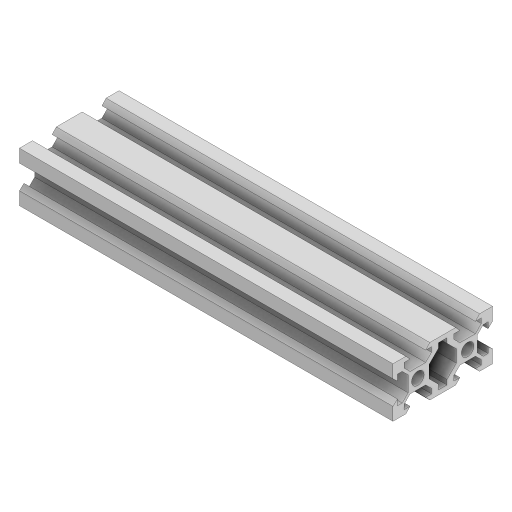
# Autodesk Inventor part: VSLOT
Saved by Autodesk Inventor 2024 (Build 280153000, 153)
## iProperties
Created: 2024-05-16
Part Number: VSLOT
Material: Generic
Document SubType Name: Modeling
Designer: Jhuliams
Density: 1 g/cm^3
Appearance: Default
Author: Jhuliams
Autodesk Inventor part; units mm, degrees
ref_plane "YZ Plane" through (0, 0, 0) normal (1, 0, 0) x (0, 1, 0)
ref_plane "XZ Plane" through (0, 0, 0) normal (0, 1, 0) x (-1, 0, 0)
ref_plane "XY Plane" through (0, 0, 0) normal (0, 0, 1) x (1, 0, 0)
sketch "Sketch1" plane through (0, 0, 0) normal (1, 0, 0) x (0, 1, 0)
  line L0 (10, 20) -> (-10, 20)
  line L1 (-10, 20) -> (-10, -20)
  line L2 (-10, -20) -> (10, -20)
  line L3 (10, -20) -> (10, 20)
  line L4 (10, 20) -> (-10, -20) construction
  line L5 (-10, 20) -> (10, -20) construction
  line L6 (0, -20) -> (0, -10) construction
  circle A0 centre (0, -10) radius 2.5
  line L7 (10, 0) -> (0, 0) construction
  circle A1 centre (0, 10) radius 2.5
  line L8 (0, 20) -> (0, 18.2) construction
  line L9 (0, 18.2) -> (3.125, 18.2)
  line L10 (0, 18.2) -> (0, 13.9)
  line L11 (0, 20) -> (4.8, 20)
  line L12 (4.8, 20) -> (3.125, 18.2)
  line L13 (0, 18.2) -> (5.5, 18.2)
  line L14 (0, 13.9) -> (3.125, 13.9)
  line L15 (5.5, 18.2) -> (5.5, 16.275)
  line L16 (3.125, 13.9) -> (5.5, 16.275)
  line L17 (3.125, 13.9) -> (8.7353, 13.9) construction
  line L18 (0, 18.2) -> (-3.125, 18.2)
  line L19 (0, 20) -> (-4.8, 20)
  line L20 (-4.8, 20) -> (-3.125, 18.2)
  line L21 (0, 18.2) -> (-5.5, 18.2)
  line L22 (0, 13.9) -> (-3.125, 13.9)
  line L23 (-5.5, 18.2) -> (-5.5, 16.275)
  line L24 (-3.125, 13.9) -> (-5.5, 16.275)
  line L25 (10, 10) -> (8.2, 10) construction
  line L26 (8.2, 10) -> (8.2, 6.875)
  line L27 (8.2, 10) -> (3.9, 10)
  line L28 (10, 10) -> (10, 5.2)
  line L29 (10, 5.2) -> (8.2, 6.875)
  line L30 (8.2, 10) -> (8.2, 4.5)
  line L31 (3.9, 10) -> (3.9, 6.875)
  line L32 (8.2, 4.5) -> (6.275, 4.5)
  line L33 (3.9, 6.875) -> (6.275, 4.5)
  line L34 (3.9, 13.125) -> (6.275, 15.5)
  line L35 (8.2, 10) -> (8.2, 15.5)
  line L36 (8.2, 15.5) -> (6.275, 15.5)
  line L37 (8.2, 10) -> (8.2, 13.125)
  line L38 (10, 10) -> (10, 14.8)
  line L39 (10, 14.8) -> (8.2, 13.125)
  line L40 (3.9, 10) -> (3.9, 13.125)
  line L41 (0, 10) -> (10, 10) construction
  line L42 (-3.9, 10) -> (-3.9, 13.125)
  line L43 (-3.9, 13.125) -> (-6.275, 15.5)
  line L44 (-8.2, 10) -> (-8.2, 15.5)
  line L45 (-8.2, 15.5) -> (-6.275, 15.5)
  line L46 (-10, 14.8) -> (-8.2, 13.125)
  line L47 (-3.9, 10) -> (-3.9, 6.875)
  line L48 (-3.9, 6.875) -> (-6.275, 4.5)
  line L49 (-8.2, 4.5) -> (-6.275, 4.5)
  line L50 (-8.2, 10) -> (-8.2, 4.5)
  line L51 (-10, 5.2) -> (-8.2, 6.875)
  line L52 (0, -20) -> (0, -18.2) construction
  line L53 (0, -18.2) -> (3.125, -18.2)
  line L54 (0, -18.2) -> (0, -13.9)
  line L55 (0, -20) -> (4.8, -20)
  line L56 (4.8, -20) -> (3.125, -18.2)
  line L57 (0, -18.2) -> (5.5, -18.2)
  line L58 (0, -13.9) -> (3.125, -13.9)
  line L59 (5.5, -18.2) -> (5.5, -16.275)
  line L60 (3.125, -13.9) -> (5.5, -16.275)
  line L61 (3.125, -13.9) -> (8.7353, -13.9) construction
  line L62 (-3.125, -13.9) -> (-5.5, -16.275)
  line L63 (0, -18.2) -> (-5.5, -18.2)
  line L64 (-5.5, -18.2) -> (-5.5, -16.275)
  line L65 (0, -18.2) -> (-3.125, -18.2)
  line L66 (0, -20) -> (-4.8, -20)
  line L67 (-4.8, -20) -> (-3.125, -18.2)
  line L68 (0, -13.9) -> (-3.125, -13.9)
  line L69 (8.2, -10) -> (8.2, -13.125)
  line L70 (3.9, -10) -> (3.9, -13.125)
  line L71 (3.9, -13.125) -> (6.275, -15.5)
  line L72 (10, -10) -> (10, -14.8)
  line L73 (8.2, -10) -> (8.2, -15.5)
  line L74 (8.2, -15.5) -> (6.275, -15.5)
  line L75 (10, -14.8) -> (8.2, -13.125)
  line L76 (3.9, -10) -> (3.9, -6.875)
  line L77 (3.9, -6.875) -> (6.275, -4.5)
  line L78 (8.2, -4.5) -> (6.275, -4.5)
  line L79 (8.2, -10) -> (3.9, -10)
  line L80 (8.2, -10) -> (8.2, -6.875)
  line L81 (8.2, -10) -> (8.2, -4.5)
  line L82 (10, -5.2) -> (8.2, -6.875)
  line L83 (10, -10) -> (10, -5.2)
  line L84 (10, -10) -> (8.2, -10) construction
  line L85 (-10, -14.8) -> (-8.2, -13.125)
  line L86 (-8.2, -10) -> (-8.2, -15.5)
  line L87 (-8.2, -15.5) -> (-6.275, -15.5)
  line L88 (-3.9, -13.125) -> (-6.275, -15.5)
  line L89 (-3.9, -10) -> (-3.9, -13.125)
  line L90 (-3.9, -10) -> (-3.9, -6.875)
  line L91 (-3.9, -6.875) -> (-6.275, -4.5)
  line L92 (-8.2, -4.5) -> (-6.275, -4.5)
  line L93 (-8.2, -10) -> (-8.2, -4.5)
  line L94 (-10, -5.2) -> (-8.2, -6.875)
  line L95 (-8.2, -4.5) -> (-8.2, 0) construction
  line L96 (-8.2, 0) -> (-8.2, 1.7)
  line L97 (-8.2, 1.7) -> (-6.275, 1.7)
  line L98 (-6.275, 1.7) -> (-2.5, 5.475)
  line L99 (-3.9, 6.875) -> (-1.2394, 4.2144) construction
  line L100 (-2.5, 5.475) -> (2.5, 5.475)
  line L101 (3.9, 6.875) -> (1.5625, 4.5375) construction
  line L102 (-6.275, 1.7) -> (13.7612, 1.7) construction
  line L103 (-6.275, 1.7) -> (13.7612, 1.7) construction
  line L104 (2.5, 5.475) -> (6.275, 1.7)
  line L105 (6.275, 1.7) -> (8.2, 1.7)
  line L106 (8.2, 1.7) -> (8.2, 0)
  line L107 (-8.2, 0) -> (-8.2, -1.7)
  line L108 (-8.2, -1.7) -> (-6.275, -1.7)
  line L109 (-6.275, -1.7) -> (-2.5, -5.475)
  line L110 (-2.5, -5.475) -> (2.5, -5.475)
  line L111 (2.5, -5.475) -> (6.275, -1.7)
  line L112 (6.275, -1.7) -> (8.2, -1.7)
  line L113 (8.2, -1.7) -> (8.2, 0)
  point P0 (10, -10)
  dimension "d0" = 20
  dimension "d1" = 40
  dimension "d2" = 10
  dimension "d3" = 5
  dimension "d4" = 10
  dimension "d5" = 1.8
  dimension "d6" = 3.125
  dimension "d7" = 4.3
  dimension "d9" = 4.8
  dimension "d11" = 5.5
  dimension "d12" = 3.125
  dimension "d13" = 45
  dimension "d14" = 1.8
  dimension "d15" = 3.125
  dimension "d16" = 4.3
  dimension "d17" = 4.8
  dimension "d18" = 5.5
  dimension "d19" = 3.125
  dimension "d20" = 1.7
  dimension "d21" = 0
  constraints: 228 end point, 68 symmetric about line, 16 point on line, 7 horizontal, 6 perpendicular, 6 vertical, 5 midpoint, 4 parallel, 2 centre point, 1 coincident, 1 collinear, 1 other
  measures "d0" distance of L2.end L1.end
  measures "d1" distance of L1.end L0.end
  measures "d2" distance of L6.start L6.end
  measures "d3" diameter of A0
  measures "d4" distance of L7.start L7.end
  measures "d5" distance of L8.start L8.end
  measures "d6" distance of L8.end L9.end
  measures "d7" distance of L8.end L10.end
  measures "d9" distance of L8.start L11.end
  measures "d11" distance of L8.end L13.end
  measures "d12" distance of L10.end L14.end
  measures "d13" angle of L17 L16
  measures "d14" distance of L38.start L37.start
  measures "d15" distance of L37.start L26.end
  measures "d16" distance of L37.start L40.start
  measures "d17" distance of L38.start L29.start
  measures "d18" distance of L37.start L32.start
  measures "d19" distance of L40.start L31.end
  measures "d20" distance of L95.end L96.end
  measures "d21" distance between parallel lines of L102 L103
extrude "Extrusion1" add sketch "Sketch1" along normal blind 150 contours L3 L39 L35 L36 L34 L40 L31 L33 L32 L30 L29 L82 L81 L78 L77 L76 L70 L71 L74 L73 L75 L2 L56 L57 L59 L60 L58 L68 L62 L64 L63 L67 L1 L85 L86 L87 L88 L89 L90 L91 L92 L93 L94 L51 L50 L49 L48 L47 L42 L43 L45 L44 L46 L0 L20 L21 L23 L24 L22 L14 L16 L15 L13 L12
body "Solid1"
